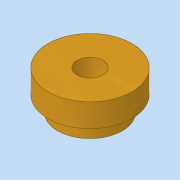
# Autodesk Inventor part: SleeveBearing2mm
Saved by Autodesk Inventor 2017 (Build 210142000, 142)
## iProperties
Created: 2017-03-04
Part Number: SleeveBearing2mm
Material: Brass, Soft Yellow, Welded
Document SubType Name: Modeling
Designer: techn
Density: 8.5 g/cm^3
Appearance: Weld - Brass
Author: techn
Autodesk Inventor part; units mm, degrees
ref_plane "YZ Plane" through (0, 0, 0) normal (1, 0, 0) x (0, 1, 0)
ref_plane "XZ Plane" through (0, 0, 0) normal (0, 1, 0) x (-1, 0, 0)
ref_plane "XY Plane" through (0, 0, 0) normal (0, 0, 1) x (1, 0, 0)
sketch "Sketch2" plane through (0, 0, 0) normal (0, 0, 1) x (1, 0, 0)
  line L0 (0, 0) -> (2.5, 0)
  line L1 (2.5, 0) -> (2.5, 1.2)
  line L2 (2.5, 1.2) -> (0, 1.2)
  line L3 (0, 1.2) -> (0, 0)
  line L4 (0, 1.2) -> (3.25, 1.2)
  line L5 (3.25, 1.2) -> (3.25, 3)
  line L6 (3.25, 3) -> (0, 3)
  line L7 (0, 3) -> (0, 1.2)
  dimension "d1" = 2.5
  dimension "d2" = 1.2
  dimension "d3" = 3.25
  dimension "d4" = 1.8
  constraints: 16 end point, 4 parallel, 2 horizontal, 2 perpendicular
  measures "d1" distance of L2.end L1.end
  measures "d2" distance of L1.end L0.end
  measures "d3" distance of L6.end L5.end
  measures "d4" distance of L5.end L4.end
revolve "Revolution1" add sketch "Sketch2" angle 360 about axis through (0, 3, 0) along (0, -1, 0)
sketch "Sketch3" plane through (0, 3, 0) normal (0, 1, 0) x (1, 0, 0)
  circle A0 centre (0, 0) radius 1
  dimension "d6" = 2
  constraints: 1 centre point, 1 coincident
  measures "d6" diameter of A0
extrude "Extrusion1" cut sketch "Sketch3" against normal through all
body "Solid1"
